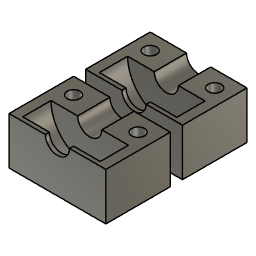
axle holder (Autodesk Fusion 360 design; units mm, degrees)
Autodesk Fusion 360 part; units mm, degrees
sketch "Sketch1" plane through (0, 0, 0) normal (0, 0, 1) x (1, 0, 0)
  line L0 (-3, 2) -> (21, 2)
  line L1 (21, 2) -> (21, -6)
  line L2 (21, -6) -> (-3, -6)
  line L3 (-3, -6) -> (-3, 2)
  dimension "d1" = 24
  dimension "d2" = 8
  constraint horizontal L0
  constraint vertical L1
  constraint horizontal L2
  constraint vertical L3
  measures "d1" distance of L0.start L0.end
  measures "d2" distance of L0.start L2.end
extrude "Extrude1" add sketch "Sketch1" along normal blind 23.4 makes body 1
extrude "Extrude2" add 1 faces at (13, -6, 7.8) along direction (0, -1, 0) blind 8 on bodies 1 bodies 1
sketch "Sketch2" plane through (0, -14, 0) normal (0, -1, 0) x (1, 0, 0)
  line L0 (-3, 0) -> (21, 0)
  line L1 (21, 0) -> (21, 23.4)
  line L2 (21, 23.4) -> (-3, 23.4)
  line L3 (-3, 23.4) -> (-3, 0)
  circle A0 centre (9, 11.7) radius 9.6
  circle A1 centre (9, 11.7) radius 3
  dimension "d7" = 19.2
  dimension "d8" = 6
  dimension "d9" = 11.7
  dimension "d10" = 12
  constraint concentric A0 A1
  measures "d7" diameter of A0
  measures "d8" diameter of A1
  measures "d9" distance of L0 A0.centre
  measures "d10" distance of L3 A0.centre
extrude "Extrude3" cut sketch "Sketch2" against normal blind 8 contours A0 | A1 bodies 1
extrude "Extrude4" add sketch "Sketch2" against normal blind 1 contours A0 bodies 1
sketch "Sketch3" plane through (0, 0, 23.4) normal (0, 0, 1) x (-1, 0, 0)
  line L0 (-21, 14) -> (-21, -2)
  line L1 (-21, -2) -> (3, -2)
  line L2 (3, -2) -> (3, 14)
  line L3 (3, 14) -> (-21, 14)
  circle A0 centre (-1, 2) radius 1.6
  circle A1 centre (-17, 2) radius 1.6
  dimension "d15" = 3.2
  dimension "d16" = 3.2
  dimension "d17" = 16
  dimension "d18" = 4
  dimension "d19" = 4
  measures "d15" diameter of A0
  measures "d16" diameter of A1
  measures "d17" distance of A0.centre A1.centre
  measures "d18" distance of L2 A0.centre
  measures "d19" distance of L1 A0.centre
extrude "Extrude5" cut sketch "Sketch3" against normal blind 25 contours A0 | A1 bodies 1
sketch "Sketch4" plane through (-3, 0, 0) normal (-1, 0, 0) x (0, -1, 0)
  line L0 (-2, 0) -> (14, 0)
  line L1 (14, 0) -> (14, 23.4)
  line L2 (14, 23.4) -> (-2, 23.4)
  line L3 (-2, 23.4) -> (-2, 0)
  line L4 (-2, 11.7) -> (14, 11.7)
  dimension "d22" = 11.7
  constraint coincident L3 L4.start
  constraint coincident L1 L4.end
  constraint perpendicular L1 L4
  measures "d22" distance of L0 L4
extrude "Extrude6" cut sketch "Sketch2" against normal blind 25 contours A1 bodies 1
split "Split1" by curves path "Sketch4" along L4 bodies 1 makes body 2 at (6.6659, -10.417, 0)
move_body "Move1" bodies 1 to x (1, 0, 0) y (0, 1, 0) z (0, 0, 1) at (0, 26, -11.7)
move_body "Move2" bodies 1 to x (-1, 0, 0) y (0, 1, 0) z (0, 0, -1) at (18, 0, 9.6)
move_body "Move3" bodies 1 to x (1, 0, 0) y (0, 1, 0) z (0, 0, 1) at (0, -7, 2.1)
